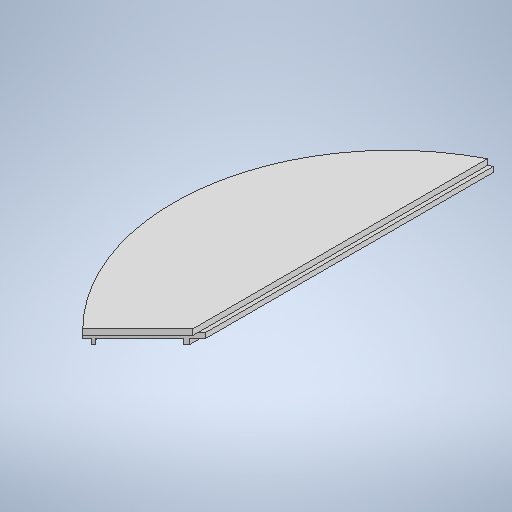
# Autodesk Inventor part: left_hull_lid
Saved by Autodesk Inventor 2025 (Build 290162000, 162)
## iProperties
Created: 2026-03-19
Part Number: left_hull_lid
Material: Generic
Document SubType Name: Modeling
Designer: Luca
Density: 1 g/cm^3
Appearance: Default
Author: Luca
Autodesk Inventor part; units mm, degrees
ref_plane "YZ Plane" through (0, 0, 0) normal (1, 0, 0) x (0, 1, 0)
ref_plane "XZ Plane" through (0, 0, 0) normal (0, 1, 0) x (-1, 0, 0)
ref_plane "XY Plane" through (0, 0, 0) normal (0, 0, 1) x (1, 0, 0)
derived "sk_reservoir.ipt"
sketch "lid_mount" plane through (0, -70, 0) normal (0, 1, 0) x (-1, 0, 0)
  line L0 (35, -68.5857) -> (35, 35) construction
  line L1 (35, 35) -> (-68.5857, 35) construction
  line L2 (38, 38) -> (-69.4029, 38) construction
  line L3 (38, -69.4029) -> (38, 38) construction
  circle A0 centre (32.5, -67.5925) radius 5
  circle A1 centre (-67.5925, 32.5) radius 5
  circle A2 centre (-67.5925, -32.5) radius 5
  circle A3 centre (-32.5, -67.5925) radius 5
  line L4 (-32.5, -67.5925) -> (32.5, -67.5925) construction
  circle A4 centre (0, 0) radius 80
  circle A5 centre (-67.5925, -32.5) radius 2.5
  circle A6 centre (32.5, -67.5925) radius 2.5
  circle A7 centre (-67.5925, 32.5) radius 2.5
  circle A8 centre (-32.5, -67.5925) radius 2.5
  circle A9 centre (67.5925, -32.5) radius 5
  circle A10 centre (-32.5, 67.5925) radius 5
  circle A11 centre (67.5925, -32.5) radius 2.5
  circle A12 centre (-32.5, 67.5925) radius 2.5
  circle A13 centre (32.5, 67.5925) radius 2.5
  circle A14 centre (32.5, 67.5925) radius 5
  circle A15 centre (67.5925, 32.5) radius 2.5
  circle A16 centre (67.5925, 32.5) radius 5
  line L5 (67.5925, 32.5) -> (67.5925, -32.5) construction
  line L6 (32.5, 67.5925) -> (-32.5, 67.5925) construction
  line L7 (0, 67.5925) -> (0, 0)
  line L8 (67.5925, 0) -> (0, 0)
  circle A17 centre (-67.5925, -32.5) radius 2.1
  circle A18 centre (32.5, 67.5925) radius 2.1
  circle A19 centre (67.5925, 32.5) radius 2.1
  circle A20 centre (32.5, -67.5925) radius 2.1
  circle A21 centre (-32.5, -67.5925) radius 2.1
  circle A22 centre (-67.5925, 32.5) radius 2.1
  circle A23 centre (-32.5, 67.5925) radius 2.1
  line L9 (33.7759, 70.2462) -> (34.6667, 72.0987) construction
  circle A24 centre (67.5925, -32.5) radius 2.1
  circle A25 centre (0, 0) radius 1.6
  line L10 (-3.4, 0) -> (-1.7, 2.9445)
  line L11 (-1.7, 2.9445) -> (1.7, 2.9445)
  line L12 (1.7, 2.9445) -> (3.4, 0)
  line L13 (3.4, 0) -> (1.7, -2.9445)
  line L14 (1.7, -2.9445) -> (-1.7, -2.9445)
  line L15 (-1.7, -2.9445) -> (-3.4, 0)
  circle A26 centre (0, 0) radius 5
  circle A27 centre (0, 0) radius 1.35
  line L16 (-67.5925, 32.5) -> (-67.5925, -32.5) construction
  point P0 (0, -67.5925)
  point P1 (-67.5925, 0)
sketch "lid" plane through (0, 0, 0) normal (0, 1, 0) x (-1, 0, 0)
  line L0 (35, 35) -> (-68.5857, 35)
  line L1 (38, 38) -> (-69.4029, 38)
  line L2 (80, 0) -> (-80, 0) construction
  circle A0 centre (0, 0) radius 80
  line L3 (0, -80) -> (0, 80) construction
  line L4 (38, -69.4029) -> (38, 38)
  line L5 (35, -68.5857) -> (35, 35)
  line L6 (0, 0) -> (56.5685, 56.5685) construction
  line L7 (36.5, 36.5) -> (36.5, -71.1881) construction
  line L8 (36.5, 36.5) -> (-71.1881, 36.5) construction
  line L9 (38, 38) -> (35, 35) construction
  line L10 (36.625, -71.1239) -> (36.625, 36.625)
  line L11 (36.375, 36.375) -> (36.375, -71.2521)
  line L12 (38, -69.4029) -> (38, -70.3989)
  line L13 (35, -68.5857) -> (35, -71.9375)
  line L14 (36.375, 36.375) -> (-71.2521, 36.375)
  line L15 (-71.1239, 36.625) -> (36.625, 36.625)
  line L16 (-69.4029, 38) -> (-70.3989, 38)
  line L17 (-68.5857, 35) -> (-71.9375, 35)
  line L18 (35, 34.8232) -> (56.6569, 56.4801)
  line L19 (32.8787, 35) -> (55.4979, 57.6193)
  line L20 (34.8232, 35) -> (56.4801, 56.6569)
  line L21 (35, 32.8787) -> (57.6193, 55.4979)
  line L22 (37.75, 37.75) -> (37.75, -70.5332)
  line L23 (35.25, -71.8153) -> (35.25, 35.25)
  line L24 (37.75, 37.75) -> (-70.5332, 37.75)
  line L25 (-71.8153, 35.25) -> (35.25, 35.25)
  line L26 (33.2322, 35) -> (55.6778, 57.4455)
  line L27 (57.4455, 55.6778) -> (35, 33.2322)
  point P0 (27, -64.5833)
  point P1 (35.25, 33.1287)
  point P2 (38, 35.8787)
  point P3 (37.75, 35.6287)
  point P4 (37.75, 35.9822)
  point P5 (38, 36.2322)
  point P6 (36.625, 36.4482)
ref_plane "lid_upper_top" through (0, 4, 0) normal (0, 1, 0) x (-1, 0, 0)
ref_plane "lid_lower_top" through (0, 1.9, 0) normal (0, 1, 0) x (-1, 0, 0)
ref_plane "lid_upper_bottom" through (0, 2, 0) normal (0, 1, 0) x (-1, 0, 0)
sketch "reservoir_lid_seal" plane through (0, 0, 0) normal (0, 1, 0) x (-1, 0, 0)
  line L0 (35, -68.5857) -> (35, 35) construction
  line L1 (35.25, -71.8153) -> (35.25, 35.25) construction
  line L2 (36.375, 36.375) -> (36.375, -71.2521) construction
  line L3 (36.5, 36.5) -> (36.5, -71.1881) construction
  line L4 (36.625, -71.1239) -> (36.625, 36.625) construction
  line L5 (37.75, 37.75) -> (37.75, -70.5332) construction
  line L6 (38, -69.4029) -> (38, 38) construction
  line L7 (0, -80) -> (0, 80) construction
  line L8 (80, 0) -> (-80, 0) construction
  line L9 (35, 35) -> (-68.5857, 35) construction
  line L10 (38, 38) -> (-69.4029, 38) construction
  line L11 (38, -69.4029) -> (38, -70.3989) construction
  line L12 (35, -68.5857) -> (35, -71.9375) construction
  line L13 (37.75, 37.75) -> (-70.5332, 37.75) construction
  line L14 (-71.1239, 36.625) -> (36.625, 36.625) construction
  line L15 (36.5, 36.5) -> (-71.1881, 36.5) construction
  line L16 (36.375, 36.375) -> (-71.2521, 36.375) construction
  line L17 (-71.8153, 35.25) -> (35.25, 35.25) construction
  line L18 (-69.4029, 38) -> (-70.3989, 38) construction
  line L19 (-68.5857, 35) -> (-71.9375, 35) construction
  line L20 (0, 0) -> (56.5685, 56.5685) construction
  line L21 (38, 38) -> (35, 35) construction
  line L22 (32.8787, 35) -> (55.4979, 57.6193)
  line L23 (33.2322, 35) -> (55.6778, 57.4455) construction
  line L24 (34.8232, 35) -> (56.4801, 56.6569) construction
  line L25 (35, 34.8232) -> (56.6569, 56.4801) construction
  line L26 (57.4455, 55.6778) -> (35, 33.2322) construction
  line L27 (35, 32.8787) -> (57.6193, 55.4979)
  circle A0 centre (-67.5925, 32.5) radius 2.1 construction
  circle A1 centre (-67.5925, 32.5) radius 2.5 construction
  circle A2 centre (-67.5925, 32.5) radius 5 construction
  line L28 (-67.5925, 32.5) -> (-67.5925, -32.5) construction
  circle A3 centre (-67.5925, -32.5) radius 2.1 construction
  circle A4 centre (-67.5925, -32.5) radius 2.5 construction
  circle A5 centre (-67.5925, -32.5) radius 5 construction
  line L29 (35, 35) -> (-68.5857, 35) construction
  line L30 (38, 38) -> (-69.4029, 38) construction
  circle A6 centre (-32.5, -67.5925) radius 5 construction
  line L31 (35, -68.5857) -> (35, 35) construction
  line L32 (38, -69.4029) -> (38, 38) construction
  circle A7 centre (0, 0) radius 80 construction
  line L33 (-32.5, -67.5925) -> (32.5, -67.5925) construction
  circle A8 centre (32.5, -67.5925) radius 5 construction
  circle A9 centre (-32.5, 67.5925) radius 2.1 construction
  circle A10 centre (-32.5, 67.5925) radius 2.5 construction
  circle A11 centre (67.5925, -32.5) radius 5 construction
  circle A12 centre (67.5925, 32.5) radius 2.1 construction
  circle A13 centre (67.5925, 32.5) radius 2.5 construction
  circle A14 centre (67.5925, 32.5) radius 5 construction
  line L34 (67.5925, 32.5) -> (67.5925, -32.5) construction
  circle A15 centre (67.5925, -32.5) radius 2.1 construction
  circle A16 centre (67.5925, -32.5) radius 2.5 construction
  circle A17 centre (-32.5, 67.5925) radius 5 construction
  circle A18 centre (32.5, 67.5925) radius 2.5 construction
  circle A19 centre (32.5, 67.5925) radius 5 construction
  line L35 (0, 67.5925) -> (0, 0) construction
  circle A20 centre (32.5, 67.5925) radius 2.1 construction
  line L36 (33.7759, 70.2462) -> (34.6667, 72.0987) construction
  line L37 (32.5, 67.5925) -> (-32.5, 67.5925) construction
  circle A21 centre (32.5, -67.5925) radius 2.5 construction
  circle A22 centre (-32.5, -67.5925) radius 2.5 construction
  circle A23 centre (32.5, -67.5925) radius 2.1 construction
  circle A24 centre (-32.5, -67.5925) radius 2.1 construction
  line L38 (67.5925, 0) -> (0, 0) construction
  line L39 (3.4, 0) -> (1.7, -2.9445) construction
  line L40 (1.7, 2.9445) -> (3.4, 0) construction
  line L41 (1.7, -2.9445) -> (-1.7, -2.9445) construction
  circle A25 centre (0, 0) radius 1.35 construction
  circle A26 centre (0, 0) radius 1.6 construction
  line L42 (-1.7, 2.9445) -> (1.7, 2.9445) construction
  line L43 (-1.7, -2.9445) -> (-3.4, 0) construction
  line L44 (-3.4, 0) -> (-1.7, 2.9445) construction
  circle A27 centre (0, 0) radius 5 construction
  circle A28 centre (67.5925, -32.5) radius 5.25
  circle A29 centre (32.5, -67.5925) radius 5.25
  circle A30 centre (-32.5, -67.5925) radius 5.25
  circle A31 centre (-67.5925, -32.5) radius 5.25
  circle A32 centre (-67.5925, 32.5) radius 5.25
  circle A33 centre (-32.5, 67.5925) radius 5.25
  circle A34 centre (32.5, 67.5925) radius 5.25
  circle A35 centre (67.5925, 32.5) radius 5.25
  circle A36 centre (0, 0) radius 5.25
  circle A37 centre (67.5925, -32.5) radius 6.25
  circle A38 centre (67.5925, 32.5) radius 6.25
  circle A39 centre (32.5, 67.5925) radius 6.25
  circle A40 centre (-32.5, 67.5925) radius 6.25
  circle A41 centre (-67.5925, 32.5) radius 6.25
  circle A42 centre (0, 0) radius 6.25
  circle A43 centre (-67.5925, -32.5) radius 6.25
  circle A44 centre (-32.5, -67.5925) radius 6.25
  circle A45 centre (32.5, -67.5925) radius 6.25
  line L45 (34.75, -72.0586) -> (34.75, 34.75)
  line L46 (34.75, 34.75) -> (-68.4324, 34.75)
  line L47 (-67.8159, 33.75) -> (33.75, 33.75)
  line L48 (33.75, 33.75) -> (33.75, -72.5323)
  arc A46 (38.25, -67.9775) -> (-67.9775, 38.25) centre (0, 0) ccw construction
  arc A47 (-68.5857, 35) -> (35, -68.5857) centre (0, 0) ccw construction
  arc A48 (-66.3253, 38.6202) -> (34.75, -68.4324) centre (0, 0) ccw
  arc A49 (-65.3373, 38.3289) -> (33.75, -67.8159) centre (0, 0) ccw
  arc A50 (38.25, -67.6905) -> (-67.6905, 38.25) centre (0, 0) ccw
  arc A51 (39.25, -65.9545) -> (-65.9545, 39.25) centre (0, 0) ccw
  line L49 (38.25, -67.6905) -> (38.25, 38.25)
  line L50 (38.25, 38.25) -> (-67.6905, 38.25)
  line L51 (-65.9545, 39.25) -> (39.25, 39.25)
  line L52 (39.25, 39.25) -> (39.25, -65.9545)
  point P0 (-67.5925, 0)
  point P1 (0, -67.5925)
  point P2 (55.3207, 53.1994)
  point P3 (66.3253, 38.6202)
  point P4 (71.5815, 27.6885)
  point P5 (71.5815, -27.6885)
  point P6 (72.3563, -28.4541)
  point P7 (71.923, 29.532)
  point P8 (67.9785, 37.7358)
  point P9 (56.028, 53.9067)
  point P10 (39.25, 37.1287)
  point P11 (38.25, 36.1287)
  point P12 (38.25, -65.143)
  point P13 (38.7472, -67.4071)
  point P14 (67.9785, -37.7358)
  point P15 (71.923, -29.532)
  point P16 (66.3253, -38.6202)
extrude "Extrusion5" add sketch "lid" along normal up to surface (1.9 mm away) from surface at 0 contours L21 L11 A0 L23 | L21 L10 A0 L11 | L21 L22 A0 L10 | L21 L4 L12 A0 L22 | L21 A0 L12 L4
extrude "Extrusion6" add sketch "lid" along normal up to surface (2.1 mm away) from surface at 1.9 contours L18 L22 L27 L10 | L27 L22 L21 L10 | L18 L4 L27 L22 | L21 L22 A0 L10 | L27 L4 L21 L22 | L18 A0 L27 L4 | L21 L4 L12 A0 L22 | L27 A0 L21 L4 | L21 A0 L12 L4
extrude "Extrusion2" add sketch "lid_mount" against normal blind 15 from surface at 70 contours A19 | A24
extrude "Extrusion8" add sketch "reservoir_lid_seal" against normal blind 2 from surface at 0 contours L27 L52 A51 A37 A50 A45 L49 | L27 A50 A38 A51 | A45 A50 L49 | A51 A35 A38 | A38 A50 A35 A51 | A51 A35 A50 A38 | A38 A50 A37 A51 | A51 A28 A50 A37 | A37 A51 A28 | A37 A50 A28 A51
chamfer "Chamfer1" distance 1 distance2 5 1 edges at (-65.4925, -15, -32.5) measured on face at (-65.9925, -15, -32.5)
chamfer "Chamfer2" distance 1 distance2 5 1 edges at (-65.4925, -15, 32.5) measured on face at (-65.9925, -15, 32.5)
chamfer "Chamfer3" distance 1 angle 45 2 edges at (-65.4925, 0, 32.5) (-65.4925, 0, -32.5)
body "Solid1"
body "Solid2"
